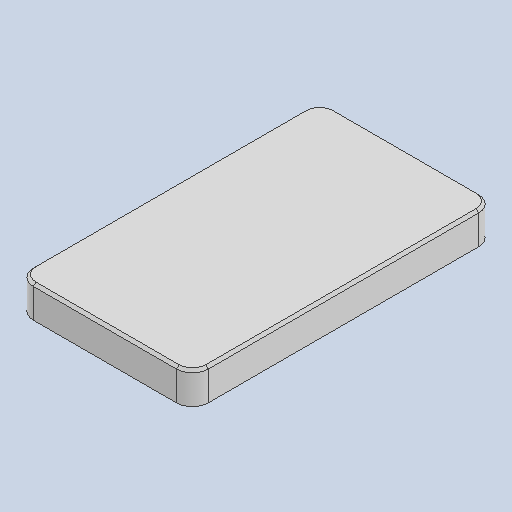
# Autodesk Inventor part: scatola_sopra
Saved by Autodesk Inventor 2022 (Build 260153000, 153)
## iProperties
Created: 2025-09-23
Part Number: scatola_sopra
Material: Generic
Document SubType Name: Modeling
Designer: 1234
Density: 1 g/cm^3
Appearance: Default
Author: 1234
Autodesk Inventor part; units mm, degrees
ref_plane "YZ Plane" through (0, 0, 0) normal (1, 0, 0) x (0, 1, 0)
ref_plane "XZ Plane" through (0, 0, 0) normal (0, 1, 0) x (-1, 0, 0)
ref_plane "XY Plane" through (0, 0, 0) normal (0, 0, 1) x (1, 0, 0)
sketch "Sketch1" plane through (0, 0, 0) normal (0, 1, 0) x (-1, 0, 0)
  line L0 (0, 0) -> (35, 0)
  line L1 (35, 0) -> (35, 75)
  line L2 (35, 75) -> (0, 75)
  line L3 (0, 75) -> (0, 0)
  line L4 (45, -10) -> (-10, -10)
  line L5 (-10, -10) -> (-10, 85)
  line L6 (-10, 85) -> (45, 85)
  line L7 (45, 85) -> (45, -10)
  line L8 (35, 0) -> (45, -10) construction
  arc A0 (40, -10) -> (45, -5) centre (40, -5) ccw
  line L9 (45, 37.5) -> (48.3975, 37.5) construction
  line L10 (17.5, 85) -> (17.5, 95.7522) construction
  arc A1 (45, 80) -> (40, 85) centre (40, 80) ccw
  arc A2 (-10, -5) -> (-5, -10) centre (-5, -5) ccw
  arc A3 (-5, 85) -> (-10, 80) centre (-5, 80) ccw
  line L11 (32, 75) -> (32, 65)
  line L12 (32, 65) -> (35, 65)
  line L13 (3, 75) -> (3, 65)
  line L14 (3, 65) -> (0, 65)
  dimension "d0" = 35
  dimension "d1" = 75
  dimension "d2" = 10
  dimension "d8" = 10
  dimension "d9" = 3
  constraints: 30 end point, 12 symmetric about line, 8 point on circle, 5 point on line, 4 centre point, 4 parallel, 3 midpoint, 3 perpendicular, 2 horizontal, 2 vertical, 1 tangent, 6 other
  measures "d0" distance of L2.end L1.end
  measures "d1" distance of L1.end L0.end
  measures "d2" distance between parallel lines of L0 L4
  measures "d8" distance between parallel lines of L2 L12
  measures "d9" distance between parallel lines of L1 L11
extrude "Extrusion1" add sketch "Sketch1" along normal blind 10 contours L3 L14 L13 L2 L11 L12 L1 L0 | L3 L2 L13 L14 | L12 L11 L2 L1 | L4 A2 L5 A3 L6 A1 L7 A0
extrude "Extrusion2" cut sketch "Sketch1" along normal blind 8 contours L3 L14 L13 L2 L11 L12 L1 L0
sketch "Sketch3" plane through (5, 0, -10) normal (0, 0, -1) x (-1, 0, 0)
  line L0 (45, 10) -> (0, 10) projected
  line L1 (22.5, 10) -> (22.5, 15.0736) construction
  line L2 (27.5, 8) -> (17.5, 8)
  line L3 (0, 10) -> (45, 10) projected
  line L4 (14.5, 5) -> (14.5, -4.5377)
  line L5 (30.5, -4.5377) -> (30.5, 5)
  line L6 (37, 0) -> (8, 0) projected
  line L7 (30.5, 0) -> (14.5, 0)
  arc A0 (30.5, 5) -> (27.5, 8) centre (27.5, 5) ccw
  arc A1 (17.5, 8) -> (14.5, 5) centre (17.5, 5) ccw
  line L8 (8, 8) -> (37, 8) projected
  point P0 (5, 0)
  point P1 (30.5, 8)
  point P2 (14.5, 8)
  dimension "d15" = 8
  dimension "d16" = 8
  dimension "d19" = 3
  constraints: 10 end point, 4 point on circle, 4 point on line, 4 tangent, 3 vertical, 2 centre point, 1 collinear, 1 equal radius, 1 midpoint, 1 parallel
  measures "d15" distance between parallel lines of L1 L5
  measures "d16" distance between parallel lines of L4 L1
  measures "d19" radius of A0
extrude "Extrusion3" [suppressed]
chamfer "Chamfer1" [suppressed]
chamfer "Chamfer2" distance 0.8 angle 45 8 edges at (-17.5, 10, -10) (-43.5355, 10, -8.5355) (-45, 10, 37.5) (-43.5355, 10, 83.5355) (-17.5, 10, 85) (8.5355, 10, 83.5355) (10, 10, 37.5) (8.5355, 10, -8.5355)
equation "\"d16\" = d15"
body "Solid1"
